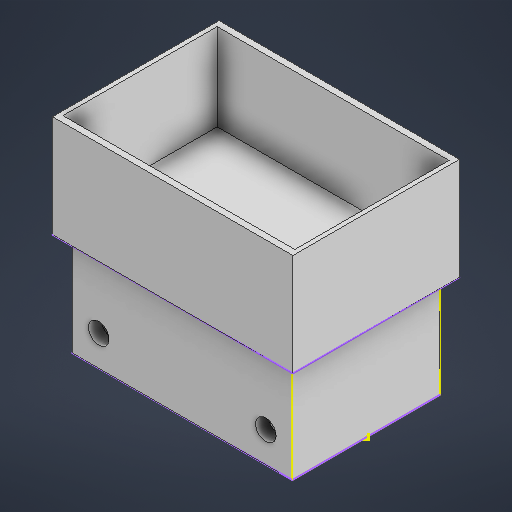
# Autodesk Inventor part: base_box
Saved by Autodesk Inventor 2026.2 (Build 302298010, 298A)
## iProperties
Created: 2026-03-24
Part Number: base_box
Material: Generic
Document SubType Name: Modeling
Designer: Srishanth Dhondy
Density: 1 g/cm^3
Appearance: Default
Mass: 1.97075 g
Surface Area: 39.9269 cm^2
Volume: 1.97075 cm^3
Author: Srishanth Dhondy
Autodesk Inventor part; units mm, degrees
ref_plane "YZ Plane" through (0, 0, 0) normal (1, 0, 0) x (0, 1, 0)
ref_plane "XZ Plane" through (0, 0, 0) normal (0, 1, 0) x (-1, 0, 0)
ref_plane "XY Plane" through (0, 0, 0) normal (0, 0, 1) x (1, 0, 0)
sketch "Sketch1" plane through (0, 0, 0) normal (0, 1, 0) x (-1, 0, 0)
  point P0 (0, 0)
sketch "Sketch2" plane through (0, 0, 0) normal (0, 1, 0) x (-1, 0, 0)
  line L0 (-10.7689, -7.215) -> (10.7689, -7.215)
  line L1 (10.7689, -7.215) -> (10.7689, 7.215)
  line L2 (10.7689, 7.215) -> (-10.7689, 7.215)
  line L3 (-10.7689, 7.215) -> (-10.7689, -7.215)
  line L4 (-10.7689, -7.215) -> (10.7689, 7.215) construction
  line L5 (10.7689, -7.215) -> (-10.7689, 7.215) construction
  line L6 (9.5058, 5.9518) -> (9.5058, -5.9518)
  line L7 (9.5058, -5.9518) -> (-9.5058, -5.9518)
  line L8 (-9.5058, -5.9518) -> (-9.5058, 5.9518)
  line L9 (-9.5058, 5.9518) -> (9.5058, 5.9518)
  point P0 (0, 0)
  constraints: 20 end point, 4 parallel, 2 midpoint, 2 perpendicular, 1 horizontal, 3 other
extrude "Extrusion1" add sketch "Sketch2" along normal blind 10
sketch "Sketch3" plane through (-10.7689, 0, 7.215) normal (0, 0, 1) x (1, 0, 0)
  circle A0 centre (2.5905, 2.9643) radius 1
  line L0 (20.2747, 10) -> (1.2632, 10) projected
  line L1 (10.7689, 10) -> (10.7689, 0)
  circle A1 centre (18.9473, 2.9643) radius 1
  dimension "d2" = 2
  constraints: 2 centre point, 2 end point, 1 midpoint, 1 perpendicular, 1 symmetric about line, 1 other
  measures "d2" diameter of A0
extrude "Extrusion2" cut sketch "Sketch3" against normal through all
extrude "Extrusion3" add sketch "Sketch2" along normal blind 1 contours L6 L7 L8 L9
sketch "Sketch4" plane through (10.7689, 0, 7.215) normal (1, 0, 0) x (0, 0, -1)
  line L0 (0, 0) -> (14.4299, 0) projected
  line L1 (14.4299, 0) -> (14.4299, 10) projected
  line L2 (0, 10) -> (14.4299, 10) projected
  line L3 (0, 0) -> (0, 10) projected
  point P0 (7.215, 0)
sketch "Sketch5" plane through (0, 10, 0) normal (0, 1, 0) x (1, 0, 0)
  line L0 (-9.5058, -5.9518) -> (-9.5058, 5.9518) projected
  line L1 (-9.5058, 5.9518) -> (9.5058, 5.9518) projected
  line L2 (9.5058, 5.9518) -> (9.5058, -5.9518) projected
  line L3 (9.5058, -5.9518) -> (-9.5058, -5.9518) projected
  line L4 (-9.7558, 6.2018) -> (-9.7558, -6.2018)
  line L5 (-9.7558, -6.2018) -> (9.7558, -6.2018)
  line L6 (9.7558, -6.2018) -> (9.7558, 6.2018)
  line L7 (9.7558, 6.2018) -> (-9.7558, 6.2018)
  point P0 (0, 0)
  dimension "d8" = 0.25
  constraints: 8 end point, 3 other
  measures "d8" distance between parallel lines of L0 L4
extrude "Extrusion4" cut sketch "Sketch5" against normal blind 0.25
sketch "Sketch6" plane through (9.7558, 10, -6.2018) normal (-1, 0, 0) x (0, 0, 1)
  line L0 (0, 0) -> (12.4036, 0) projected
  line L1 (0, 0) -> (0, -0.25) projected
  line L2 (0, -0.25) -> (12.4036, -0.25) projected
  line L3 (12.4036, 0) -> (12.4036, -0.25) projected
  point P0 (6.2018, -10)
sketch "Sketch7" plane through (10.7689, 0, 7.215) normal (1, 0, 0) x (0, 0, -1)
  line L0 (0, 10) -> (14.4299, 10) projected
  line L1 (1.0132, 10) -> (1.0132, 9.75) projected
  line L2 (13.4167, 10) -> (1.0132, 10) projected
  line L3 (1.0132, 10) -> (13.4167, 10)
  line L4 (1.0132, 10) -> (13.4167, 10)
  line L5 (1.0132, 10) -> (1.0132, 9.75)
  line L6 (1.0132, 9.75) -> (13.4167, 9.75)
  line L7 (13.4167, 9.75) -> (13.4167, 10)
  line L8 (13.4167, 10) -> (1.0132, 10)
  line L9 (1.0132, 10) -> (13.4167, 10)
  line L10 (13.4167, 10) -> (13.4167, 9.75)
  line L11 (13.4167, 9.75) -> (1.0132, 9.75)
  line L12 (1.0132, 9.75) -> (1.0132, 10)
  point P0 (7.215, 0)
  dimension "d11" = 0.25
  constraints: 20 end point, 3 parallel, 2 collinear, 2 horizontal, 2 perpendicular
  measures "d11" distance of L1.start L1.end
extrude "Extrusion5" cut sketch "Sketch7" against normal up to surface (1.0132 mm away)
sketch "Sketch8" plane through (0, 10, 0) normal (0, 1, 0) x (1, 0, 0)
  line L0 (11.7647, -8.1506) -> (-11.7647, -8.1506)
  line L1 (-11.7647, -8.1506) -> (-11.7647, 8.1506)
  line L2 (-11.7647, 8.1506) -> (11.7647, 8.1506)
  line L3 (11.7647, 8.1506) -> (11.7647, -8.1506)
  line L4 (11.7647, -8.1506) -> (-11.7647, 8.1506) construction
  line L5 (-11.7647, -8.1506) -> (11.7647, 8.1506) construction
  line L6 (11.3506, -7.5482) -> (-11.3506, -7.5482)
  line L7 (-11.3506, -7.5482) -> (-11.3506, 7.5482)
  line L8 (-11.3506, 7.5482) -> (11.3506, 7.5482)
  line L9 (11.3506, 7.5482) -> (11.3506, -7.5482)
  line L10 (11.3506, -7.5482) -> (-11.3506, 7.5482) construction
  line L11 (-11.3506, -7.5482) -> (11.3506, 7.5482) construction
  point P0 (0, 0)
  constraints: 24 end point, 4 midpoint, 4 parallel, 2 horizontal, 2 perpendicular
extrude "Extrusion6" add sketch "Sketch8" along normal blind 10
sketch "Sketch9" plane through (0, 10, 0) normal (0, 1, 0) x (1, 0, 0)
  line L0 (-9.7558, 6.2018) -> (10.7689, 6.2018) projected
  line L1 (10.7689, 6.2018) -> (10.7689, 7.215) projected
  line L2 (10.7689, 7.215) -> (-10.7689, 7.215) projected
  line L3 (-10.7689, 7.215) -> (-10.7689, -7.215) projected
  line L4 (-10.7689, -7.215) -> (10.7689, -7.215) projected
  line L5 (10.7689, -7.215) -> (10.7689, -6.2018) projected
  line L6 (10.7689, -6.2018) -> (-9.7558, -6.2018) projected
  line L7 (-9.7558, -6.2018) -> (-9.7558, 6.2018) projected
  line L8 (10.7689, -7.215) -> (-10.7689, -7.215)
  line L9 (-10.7689, -7.215) -> (-10.7689, 7.215)
  line L10 (-10.7689, 7.215) -> (10.7689, 7.215)
  line L11 (10.7689, 7.215) -> (10.7689, -7.215)
  line L12 (10.7689, -7.215) -> (-10.7689, 7.215) construction
  line L13 (-10.7689, -7.215) -> (10.7689, 7.215) construction
  point P0 (0, 0)
  constraints: 12 end point, 2 midpoint, 2 parallel, 1 horizontal, 1 perpendicular
extrude "Extrusion7" add sketch "Sketch8" along normal blind 1.5 contours L6 L7 L8 L9
body "Solid1"
